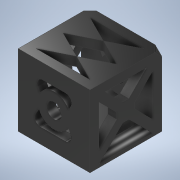
# Autodesk Inventor part: top-idler V2
Saved by Autodesk Inventor 2020.4 (Build 244396000, 396)
## iProperties
Created: 2021-04-07
Part Number: top-idler V2
Material: ABS Plastic
Document SubType Name: Modeling
Designer: AOB
Mass: 5.78199 g
Surface Area: 56.391 cm^2
Volume: 5.45471 cm^3
Density: 1.06 g/cm^3
Appearance: Glossy - Black
Author: AOB
Autodesk Inventor part; units mm, degrees
ref_plane "YZ Plane" through (0, 0, 0) normal (1, 0, 0) x (0, 1, 0)
ref_plane "XZ Plane" through (0, 0, 0) normal (0, 1, 0) x (-1, 0, 0)
ref_plane "XY Plane" through (0, 0, 0) normal (0, 0, 1) x (1, 0, 0)
sketch "Sketch1" plane through (0, 0, 0) normal (0, 0, 1) x (1, 0, 0)
  line L0 (0, 0) -> (18, 0) construction
  line L1 (18, 0) -> (18, -18) construction
  line L2 (18, -18) -> (0, -18) construction
  line L3 (0, -18) -> (0, 0) construction
  line L4 (-3, 3) -> (21, 3)
  line L5 (21, 3) -> (21, -21)
  line L6 (21, -21) -> (-3, -21)
  line L7 (-3, -21) -> (-3, 3)
  dimension "d0" = 18
  dimension "d1" = 18
  dimension "d2" = 24
  dimension "d3" = 24
  dimension "d4" = 3
  dimension "d5" = 3
  constraints: 16 end point, 4 parallel, 2 horizontal, 2 perpendicular
  measures "d0" distance of L0.start L0.end
  measures "d1" distance of L0.end L1.end
  measures "d2" distance of L5.end L6.end
  measures "d3" distance of L4.end L5.end
  measures "d4" distance between parallel lines of L4 L0
  measures "d5" distance between parallel lines of L7 L3
extrude "Extrusion1" add sketch "Sketch1" along normal blind 24
shell "Shell1" thickness 3 removed faces 0
sketch "Sketch3" plane through (0, 0, 24) normal (0, 0, 1) x (1, 0, 0)
  line L0 (21, 3) -> (-3, 3) projected
  line L1 (-3, 3) -> (-3, -21) projected
  line L2 (21, 3) -> (-3, -21)
  line L3 (-3, -21) -> (21, -21) projected
  line L4 (9, -9) -> (21, -21)
  line L5 (0, -18) -> (18, -18) construction
  line L6 (9, -18) -> (9, -16) construction
  line L7 (9, 0) -> (9, -2) construction
  line L8 (16, -2) -> (9, -16)
  line L9 (9, -16) -> (2, -2)
  line L10 (2, -2) -> (16, -2)
  line L11 (9, -2) -> (1, -16)
  line L12 (1, -16) -> (16, -16)
  line L13 (9, -2) -> (16, -16)
  point P0 (0, 0)
  point P1 (12.5, -9)
  point P2 (5.2667, -8.5333)
  dimension "d16" = 2
  dimension "d17" = 2
  constraints: 20 end point, 2 midpoint, 2 parallel, 2 point on line, 2 vertical
  measures "d16" distance of L6.start L6.end
  measures "d17" distance of L7.start L7.end
extrude "Extrusion3" cut sketch "Sketch3" against normal blind 10 contours L8 L13 L2 | L2 L13 L10 | L13 L8 L4 L2 | L2 L9 L11 L13 | L13 L4 L8 | L11 L9 L10 | L12 L11 L9 L2 | L2 L9 L12 | L4 L8 L9 L2 | L4 L12 L8
fillet "Fillet2" radius 2 4 edges at (2, -2, 22.5) (16, -2, 22.5) (16, -16, 22.5) (1, -16, 22.5)
sketch "Sketch6" plane through (0, 0, 24) normal (0, 0, 1) x (1, 0, 0)
  circle A0 centre (9, -9) radius 5.5
  circle A1 centre (9, -9) radius 2.5
  point P0 (0, 0)
  dimension "d26" = 11
  dimension "d27" = 5
  constraints: 2 centre point, 1 coincident
  measures "d26" diameter of A0
  measures "d27" diameter of A1
extrude "Extrusion5" add sketch "Sketch6" against normal blind 3
ref_plane "Work Plane1" through (0, 0, 12) normal (0, 0, -1) x (-1, 0, 0)
mirror "Mirror1" about plane through (0, 0, 12) normal (0, 0, -1) of "Extrusion5", "Fillet2", "Extrusion3"
sketch "Sketch7" plane through (-3, -21, 0) normal (-1, 0, 0) x (0, 0, 1)
  line L0 (5, 19) -> (19, 19)
  line L1 (19, 19) -> (19, 5)
  line L2 (19, 5) -> (5, 5)
  line L3 (5, 5) -> (5, 19)
  line L4 (0, 24) -> (24, 24) projected
  line L5 (0, 24) -> (0, 0) projected
  line L6 (2, 24) -> (0, 22)
  line L7 (0, 22) -> (22, 0)
  line L8 (0, 0) -> (24, 0) projected
  line L9 (24, 0) -> (24, 24) projected
  line L10 (24, 2) -> (2, 24)
  line L11 (3, 21) -> (21, 21) projected
  line L12 (3, 21) -> (3, 3) projected
  line L13 (21, 21) -> (21, 3) projected
  line L14 (3, 3) -> (21, 3) projected
  line L15 (7, 17) -> (17, 17)
  line L16 (17, 17) -> (17, 7)
  line L17 (17, 7) -> (7, 7)
  line L18 (7, 7) -> (7, 17)
  line L19 (9, 15) -> (15, 15)
  line L20 (15, 15) -> (15, 9)
  line L21 (15, 9) -> (9, 9)
  line L22 (9, 9) -> (9, 15)
  line L23 (11, 13) -> (13, 13)
  line L24 (13, 13) -> (13, 11)
  line L25 (13, 11) -> (11, 11)
  line L26 (11, 11) -> (11, 13)
  line L27 (24, 22) -> (2, 0)
  line L28 (0, 2) -> (22, 24)
  point P0 (15, 11)
  point P1 (17, 9)
  point P2 (9, 17)
  point P3 (11, 15)
  point P4 (9, 13)
  point P5 (7, 15)
  point P6 (15, 7)
  point P7 (13, 9)
  point P8 (19, 3)
  point P9 (17, 5)
  point P10 (5, 17)
  point P11 (3, 19)
  point P12 (21, 5)
  point P13 (5, 21)
  point P14 (7, 19)
  point P15 (19, 7)
  point P16 (5, 7)
  point P17 (3, 5)
  point P18 (5, 3)
  point P19 (7, 5)
  point P20 (9, 11)
  point P21 (7, 9)
  point P22 (9, 7)
  point P23 (11, 9)
  point P24 (15, 17)
  point P25 (13, 15)
  point P26 (15, 13)
  point P27 (17, 15)
  point P28 (19, 21)
  point P29 (17, 19)
  point P30 (19, 17)
  point P31 (21, 19)
  dimension "d30" = 14
  dimension "d31" = 14
  dimension "d33" = 2
  dimension "d34" = 2
  constraints: 42 end point, 9 parallel, 4 horizontal, 4 perpendicular, 4 point on line
  measures "d30" distance of L1.end L2.end
  measures "d31" distance of L0.end L1.end
  measures "d33" distance between parallel lines of L14 L2
  measures "d34" distance between parallel lines of L1 L13
extrude "Extrusion6" cut sketch "Sketch7" against normal through all contours L10 L11 L28 L0 | L0 L28 L15 L10 | L7 L18 L28 L3 | L3 L28 L12 L7 | L15 L28 L19 L10 | L7 L22 L28 L18 | L27 L13 L10 L1 | L1 L10 L16 L27 | L27 L17 L7 L2 | L2 L7 L14 L27 | L16 L10 L20 L27 | L27 L21 L7 L17
sketch "Sketch8" plane through (0, 0, 0) normal (0, 0, -1) x (-1, 0, 0)
  line L0 (-21, 3) -> (3, 3) projected
  line L1 (3, 3) -> (1, 3)
  point P0 (0, 0)
  dimension "d39" = 2
  constraints: 2 end point, 1 point on line
  measures "d39" distance of L0.end L1.end
ref_plane "Work Plane2" through (-1, 3, 0) normal (0.5773503, -0.5773503, 0.5773503) x (-0.7071068, 0, 0.7071068)
split "Split1" plane through (-1, 3, 0) removes the side toward (-0.5773503, 0.5773503, -0.5773503)
fillet "Fillet5" radius 0.3 3 edges at (-2, 3, 1) (-3, 2, 1) (-2, 2, 0)
fillet "Fillet6" radius 2 2 edges at (-3, -18, 12) (21, -18, 12) inverted yes
fillet "Fillet7" radius 2 2 edges at (-1, -18, 12) (19, -18, 12)
sketch "Sketch9" plane through (0, 0, 0) normal (0, 0, -1) x (-1, 0, 0)
  line L0 (-21, 3) -> (0.7804, 3) projected
  line L1 (-21, -21) -> (-21, 3) projected
  line L2 (-21, 3) -> (-19, 3)
  line L3 (-21, 3) -> (-21, 1)
  line L4 (-21, -21) -> (-21, 3) projected
  point P0 (0, 0)
  dimension "d45" = 2
  dimension "d46" = 2
  constraints: 4 end point, 2 point on line
  measures "d45" distance of L0.start L2.end
  measures "d46" distance of L0.start L3.end
sketch "Sketch10" plane through (21, -21, 0) normal (1, 0, 0) x (0, 0, -1)
  line L0 (0, 24) -> (-24, 24) projected
  line L1 (0, 24) -> (-2, 24)
  point P0 (0, 21)
  dimension "d47" = 2
  constraints: 2 end point, 1 point on line
  measures "d47" distance of L0.start L1.end
ref_plane "Work Plane3" through (21, 3, 2) normal (0.5773503, 0.5773503, -0.5773503) x (0, -0.7071068, -0.7071068)
split "Split2" plane through (21, 3, 2) removes the side toward (0.5773503, 0.5773503, -0.5773503)
fillet "Fillet10" radius 0.5 3 edges at (20, 2, 0) (20, 3, 1) (21, 2, 1)
sketch "Sketch11" plane through (-3, 3, 24) normal (0, 1, 0) x (1, 0, 0)
  line L0 (24, 0) -> (0, 0) projected
  line L1 (2.2196, 24) -> (0, 24) projected
  line L2 (0, 21.7804) -> (0, 0) projected
  line L3 (21, 21) -> (3, 21) projected
  line L4 (21, 3) -> (3, 3) projected
  line L5 (21, 13) -> (21, 19) projected
  line L6 (21, 5) -> (21, 11) projected
  line L7 (21, 21) -> (21, 19) projected
  line L8 (21, 11) -> (21, 13) projected
  line L9 (21, 5) -> (21, 3) projected
  line L10 (3, 13) -> (3, 11) projected
  line L11 (21, 3) -> (3, 12)
  line L12 (21, 21) -> (3, 12)
  line L13 (3, 21) -> (3, 15) projected
  line L14 (3, 21) -> (21, 12)
  line L15 (21, 13) -> (21, 11) projected
  line L16 (3, 3) -> (3, 9) projected
  line L17 (3, 3) -> (21, 12)
  line L18 (3, 19) -> (3, 13) projected
  line L19 (3, 11) -> (3, 5) projected
  point P0 (3, 24)
  point P1 (12, 7.5)
  point P2 (12, 16.5)
  constraints: 8 end point, 2 midpoint
extrude "Extrusion8" cut sketch "Sketch11" against normal blind 3 contours L12 L14 L3 | L14 L17 L11 L12 | L11 L4 L17
sketch "Sketch12" plane through (-3, -21, 0) normal (0, -1, 0) x (1, 0, 0)
  line L0 (3.4641, 3) -> (20.5359, 3) projected
  line L1 (20.5359, 3) -> (20.5359, 21) projected
  line L2 (3.4641, 21) -> (3.4641, 3) projected
  line L3 (3.4641, 21) -> (20.5359, 21) projected
  line L4 (20.5359, 3) -> (17.5359, 3)
  line L5 (21, 3) -> (3, 3)
  line L6 (17.5359, 3) -> (17.5359, 21)
  line L7 (3.4641, 3) -> (6.4641, 3)
  line L8 (7.4464, 3) -> (5.4464, 3) projected
  line L9 (6.4641, 3) -> (6.4641, 21)
  point P0 (3, 0)
  point P1 (5.7099, 3)
  point P2 (17.5359, 3)
  dimension "d51" = 3
  dimension "d52" = 3
  constraints: 10 end point, 4 point on line, 2 perpendicular
  measures "d51" distance of L0.end L4.end
  measures "d52" distance of L0.start L7.end
extrude "Extrusion9" cut sketch "Sketch12" against normal blind 3 contours L2 L3 L9 L0 | L3 L1 L0 L6
body "Solid1"
